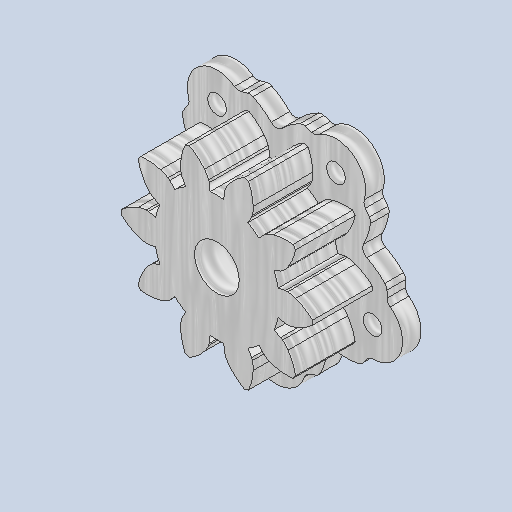
# Autodesk Inventor part: m2z10t8
Saved by Autodesk Inventor 2023 (Build 270158030, 158C)
## iProperties
Created: 2022-06-25
Part Number: m2z10t8
Material: アルミニウム 7075
Document SubType Name: Modeling
Designer: muzho
Density: 2.81 g/cm^3
Appearance: サテン - ブラシ仕上げ 重厚
Mass: 12.0512 g
Surface Area: 29.3851 cm^2
Volume: 4.2887 cm^3
Author: muzho
Autodesk Inventor part; units mm, degrees
ref_plane "YZ Plane" through (0, 0, 0) normal (1, 0, 0) x (0, 1, 0)
ref_plane "XZ Plane" through (0, 0, 0) normal (0, 1, 0) x (-1, 0, 0)
ref_plane "XY Plane" through (0, 0, 0) normal (0, 0, 1) x (1, 0, 0)
sketch "スケッチ3" plane through (0, 0, 0) normal (0, 0, 1) x (1, 0, 0)
  arc A0 (1.1108, 9.6353) -> (1.0261, 9.3407) centre (2.3523, 9.119) ccw
  arc A1 (1.6629, 10.5811) -> (1.1108, 9.6353) centre (4.6273, 8.2165) ccw
  arc A2 (3.6967, 12.3097) -> (1.6629, 10.5811) centre (7.0908, 6.2556) ccw
  arc A3 (-4.7648, 8.448) -> (-4.6602, 8.16) centre (-3.4569, 8.7601) ccw
  arc A4 (-4.8741, 9.5378) -> (-4.7648, 8.448) centre (-1.0859, 9.3672) ccw
  arc A5 (-4.2448, 12.1316) -> (-4.8741, 9.5378) centre (2.0596, 9.2288) ccw
  arc A6 (-8.8205, 4.0339) -> (-8.5665, 3.8624) centre (-7.9458, 5.0551) ccw
  arc A7 (-9.5494, 4.8513) -> (-8.8205, 4.0339) centre (-6.3844, 6.9399) ccw
  arc A8 (-10.5649, 7.3197) -> (-9.5494, 4.8513) centre (-3.7583, 8.6769) ccw
  arc A9 (-9.507, -1.921) -> (-9.2007, -1.9105) centre (-9.3996, -0.5807) ccw
  arc A10 (-10.5771, -1.6882) -> (-9.507, -1.921) centre (-9.2443, 1.8618) ccw
  arc A11 (-12.8496, -0.2881) -> (-10.5771, -1.6882) centre (-8.1406, 4.8107) ccw
  arc A12 (-6.5621, -7.1422) -> (-6.3205, -6.9537) centre (-7.2631, -5.9948) ccw
  arc A13 (-7.5648, -7.5828) -> (-6.5621, -7.1422) centre (-8.5731, -3.9274) ccw
  arc A14 (-10.2262, -7.7859) -> (-7.5648, -7.5828) centre (-9.4136, -0.893) ccw
  arc A15 (-1.1108, -9.6353) -> (-1.0261, -9.3407) centre (-2.3523, -9.119) ccw
  arc A16 (-1.6629, -10.5811) -> (-1.1108, -9.6353) centre (-4.6273, -8.2165) ccw
  arc A17 (-3.6967, -12.3097) -> (-1.6629, -10.5811) centre (-7.0908, -6.2556) ccw
  arc A18 (4.7648, -8.448) -> (4.6602, -8.16) centre (3.4569, -8.7601) ccw
  arc A19 (4.8741, -9.5378) -> (4.7648, -8.448) centre (1.0859, -9.3672) ccw
  arc A20 (4.2448, -12.1316) -> (4.8741, -9.5378) centre (-2.0596, -9.2288) ccw
  arc A21 (8.8205, -4.0339) -> (8.5665, -3.8624) centre (7.9458, -5.0551) ccw
  arc A22 (9.5494, -4.8513) -> (8.8205, -4.0339) centre (6.3844, -6.9399) ccw
  arc A23 (10.5649, -7.3197) -> (9.5494, -4.8513) centre (3.7583, -8.6769) ccw
  arc A24 (9.507, 1.921) -> (9.2007, 1.9105) centre (9.3996, 0.5807) ccw
  arc A25 (10.5771, 1.6882) -> (9.507, 1.921) centre (9.2443, -1.8618) ccw
  arc A26 (12.8496, 0.2881) -> (10.5771, 1.6882) centre (8.1406, -4.8107) ccw
  arc A27 (6.5621, 7.1422) -> (6.3205, 6.9537) centre (7.2631, 5.9948) ccw
  arc A28 (7.5648, 7.5828) -> (6.5621, 7.1422) centre (8.5731, 3.9274) ccw
  arc A29 (10.2262, 7.7859) -> (7.5648, 7.5828) centre (9.4136, 0.893) ccw
  arc A30 (-1.0261, 9.3407) -> (-1.1108, 9.6353) centre (-2.3523, 9.119) ccw
  arc A31 (-1.1108, 9.6353) -> (-1.6629, 10.5811) centre (-4.6273, 8.2165) ccw
  arc A32 (-1.6629, 10.5811) -> (-3.6967, 12.3097) centre (-7.0908, 6.2556) ccw
  arc A33 (-6.3205, 6.9537) -> (-6.5621, 7.1422) centre (-7.2631, 5.9948) ccw
  arc A34 (-6.5621, 7.1422) -> (-7.5648, 7.5828) centre (-8.5731, 3.9274) ccw
  arc A35 (-7.5648, 7.5828) -> (-10.2262, 7.7859) centre (-9.4136, 0.893) ccw
  arc A36 (-9.2007, 1.9105) -> (-9.507, 1.921) centre (-9.3996, 0.5807) ccw
  arc A37 (-9.507, 1.921) -> (-10.5771, 1.6882) centre (-9.2443, -1.8618) ccw
  arc A38 (-10.5771, 1.6882) -> (-12.8496, 0.2881) centre (-8.1406, -4.8107) ccw
  arc A39 (-8.5665, -3.8624) -> (-8.8205, -4.0339) centre (-7.9458, -5.0551) ccw
  arc A40 (-8.8205, -4.0339) -> (-9.5494, -4.8513) centre (-6.3844, -6.9399) ccw
  arc A41 (-9.5494, -4.8513) -> (-10.5649, -7.3197) centre (-3.7583, -8.6769) ccw
  arc A42 (-4.6602, -8.16) -> (-4.7648, -8.448) centre (-3.4569, -8.7601) ccw
  arc A43 (-4.7648, -8.448) -> (-4.8742, -9.5338) centre (-1.0859, -9.3672) ccw
  arc A44 (-4.8742, -9.5338) -> (-4.2448, -12.1316) centre (2.0596, -9.2288) ccw
  arc A45 (1.0261, -9.3407) -> (1.1108, -9.6353) centre (2.3523, -9.119) ccw
  arc A46 (1.1108, -9.6353) -> (1.6629, -10.5811) centre (4.6273, -8.2165) ccw
  arc A47 (1.6629, -10.5811) -> (3.6967, -12.3097) centre (7.0908, -6.2556) ccw
  arc A48 (6.3205, -6.9537) -> (6.5621, -7.1422) centre (7.2631, -5.9948) ccw
  arc A49 (6.5621, -7.1422) -> (7.5648, -7.5828) centre (8.5731, -3.9274) ccw
  arc A50 (7.5648, -7.5828) -> (10.2262, -7.7859) centre (9.4136, -0.893) ccw
  arc A51 (9.2007, -1.9105) -> (9.507, -1.921) centre (9.3996, -0.5807) ccw
  arc A52 (9.507, -1.921) -> (10.5771, -1.6882) centre (9.2443, 1.8618) ccw
  arc A53 (10.5771, -1.6882) -> (12.8496, -0.2881) centre (8.1406, 4.8107) ccw
  arc A54 (8.5665, 3.8624) -> (8.8205, 4.0339) centre (7.9458, 5.0551) ccw
  arc A55 (8.8205, 4.0339) -> (9.5494, 4.8513) centre (6.3844, 6.9399) ccw
  arc A56 (9.5494, 4.8513) -> (10.5649, 7.3197) centre (3.7583, 8.6769) ccw
  arc A57 (4.6602, 8.16) -> (4.7648, 8.448) centre (3.4569, 8.7601) ccw
  arc A58 (4.7648, 8.448) -> (4.8741, 9.5378) centre (1.0859, 9.3672) ccw
  arc A59 (4.8741, 9.5378) -> (4.2448, 12.1316) centre (-2.0596, 9.2288) ccw
  arc A60 (0.9173, 8.3498) -> (-0.9173, 8.3498) centre (0, 0) ccw
  arc A61 (-4.1658, 7.2943) -> (-5.65, 6.2159) centre (0, 0) ccw
  arc A62 (-7.6576, 3.4526) -> (-8.2246, 1.7078) centre (0, 0) ccw
  arc A63 (-8.2246, -1.7078) -> (-7.6576, -3.4526) centre (0, 0) ccw
  arc A64 (-5.65, -6.2159) -> (-4.1658, -7.2943) centre (0, 0) ccw
  arc A65 (-0.9173, -8.3498) -> (0.9173, -8.3498) centre (0, 0) ccw
  arc A66 (4.1658, -7.2943) -> (5.65, -6.2159) centre (0, 0) ccw
  arc A67 (7.6576, -3.4526) -> (8.2246, -1.7078) centre (0, 0) ccw
  arc A68 (8.2246, 1.7078) -> (7.6576, 3.4526) centre (0, 0) ccw
  arc A69 (5.65, 6.2159) -> (4.1658, 7.2943) centre (0, 0) ccw
  arc A70 (-3.6967, 12.3097) -> (-4.2448, 12.1316) centre (0, 0) ccw
  arc A71 (-10.2262, 7.7859) -> (-10.5649, 7.3197) centre (0, 0) ccw
  arc A72 (-12.8496, 0.2881) -> (-12.8496, -0.2881) centre (0, 0) ccw
  arc A73 (-10.5649, -7.3197) -> (-10.2262, -7.7859) centre (0, 0) ccw
  arc A74 (-4.2448, -12.1316) -> (-3.6967, -12.3097) centre (0, 0) ccw
  arc A75 (3.6967, -12.3097) -> (4.2448, -12.1316) centre (0, 0) ccw
  arc A76 (10.2262, -7.7859) -> (10.5649, -7.3197) centre (0, 0) ccw
  arc A77 (12.8496, -0.2881) -> (12.8496, 0.2881) centre (0, 0) ccw
  arc A78 (10.5649, 7.3197) -> (10.2262, 7.7859) centre (0, 0) ccw
  arc A79 (4.2448, 12.1316) -> (3.6967, 12.3097) centre (0, 0) ccw
  line L0 (0.9173, 8.3498) -> (1.0261, 9.3407)
  line L1 (-4.1658, 7.2943) -> (-4.6602, 8.16)
  line L2 (-7.6576, 3.4526) -> (-8.5665, 3.8624)
  line L3 (-8.2246, -1.7078) -> (-9.2007, -1.9105)
  line L4 (-5.65, -6.2159) -> (-6.3205, -6.9537)
  line L5 (-0.9173, -8.3498) -> (-1.0261, -9.3407)
  line L6 (4.1658, -7.2943) -> (4.6602, -8.16)
  line L7 (7.6576, -3.4526) -> (8.5665, -3.8624)
  line L8 (8.2246, 1.7078) -> (9.2007, 1.9105)
  line L9 (5.65, 6.2159) -> (6.3205, 6.9537)
  line L10 (-0.9173, 8.3498) -> (-1.0261, 9.3407)
  line L11 (-5.65, 6.2159) -> (-6.3205, 6.9537)
  line L12 (-8.2246, 1.7078) -> (-9.2007, 1.9105)
  line L13 (-7.6576, -3.4526) -> (-8.5665, -3.8624)
  line L14 (-4.1658, -7.2943) -> (-4.6602, -8.16)
  line L15 (0.9173, -8.3498) -> (1.0261, -9.3407)
  line L16 (5.65, -6.2159) -> (6.3205, -6.9537)
  line L17 (8.2246, -1.7078) -> (9.2007, -1.9105)
  line L18 (7.6576, 3.4526) -> (8.5665, 3.8624)
  line L19 (4.1658, 7.2943) -> (4.6602, 8.16)
  circle A80 centre (0, 0) radius 3
  point P0 (0, 0)
  dimension "d3" = 6
  constraints: 160 point on circle, 81 centre point, 40 end point, 1 coincident
  measures "d3" diameter of A80
extrude "押し出し2" add sketch "スケッチ3" along normal blind 8
sketch "スケッチ4" plane through (0, 0, 0) normal (0, 0, -1) x (-1, 0, 0)
  line L0 (-4.1658, 7.2943) -> (-4.6602, 8.16) projected
  arc A0 (-4.1658, 7.2943) -> (-5.65, 6.2159) centre (0, 0) ccw projected
  line L1 (-6.3205, 6.9537) -> (-5.65, 6.2159) projected
  arc A1 (-6.3205, 6.9537) -> (-6.5621, 7.1422) centre (-7.2631, 5.9948) ccw projected
  arc A2 (-6.5621, 7.1422) -> (-7.5648, 7.5828) centre (-8.5731, 3.9274) ccw projected
  arc A3 (-7.5648, 7.5828) -> (-10.2262, 7.7859) centre (-9.4136, 0.893) ccw projected
  arc A4 (-10.2262, 7.7859) -> (-10.5649, 7.3197) centre (0, 0) ccw projected
  arc A5 (-10.5649, 7.3197) -> (-9.5494, 4.8513) centre (-3.7583, 8.6769) ccw projected
  arc A6 (-9.5494, 4.8513) -> (-8.8205, 4.0339) centre (-6.3844, 6.9399) ccw projected
  arc A7 (-8.8205, 4.0339) -> (-8.5665, 3.8624) centre (-7.9458, 5.0551) ccw projected
  line L2 (-7.6576, 3.4526) -> (-8.5665, 3.8624) projected
  arc A8 (-7.6576, 3.4526) -> (-8.2246, 1.7078) centre (0, 0) ccw projected
  line L3 (-9.2007, 1.9105) -> (-8.2246, 1.7078) projected
  arc A9 (-9.2007, 1.9105) -> (-9.507, 1.921) centre (-9.3996, 0.5807) ccw projected
  arc A10 (-9.507, 1.921) -> (-10.5771, 1.6882) centre (-9.2443, -1.8618) ccw projected
  arc A11 (-10.5771, 1.6882) -> (-12.8496, 0.2881) centre (-8.1406, -4.8107) ccw projected
  arc A12 (-12.8496, 0.2881) -> (-12.8496, -0.2881) centre (0, 0) ccw projected
  arc A13 (-12.8496, -0.2881) -> (-10.5771, -1.6882) centre (-8.1406, 4.8107) ccw projected
  arc A14 (-10.5771, -1.6882) -> (-9.507, -1.921) centre (-9.2443, 1.8618) ccw projected
  arc A15 (-9.507, -1.921) -> (-9.2007, -1.9105) centre (-9.3996, -0.5807) ccw projected
  line L4 (-8.2246, -1.7078) -> (-9.2007, -1.9105) projected
  arc A16 (-8.2246, -1.7078) -> (-7.6576, -3.4526) centre (0, 0) ccw projected
  line L5 (-8.5665, -3.8624) -> (-7.6576, -3.4526) projected
  arc A17 (-8.5665, -3.8624) -> (-8.8205, -4.0339) centre (-7.9458, -5.0551) ccw projected
  arc A18 (-8.8205, -4.0339) -> (-9.5494, -4.8513) centre (-6.3844, -6.9399) ccw projected
  arc A19 (-9.5494, -4.8513) -> (-10.5649, -7.3197) centre (-3.7583, -8.6769) ccw projected
  arc A20 (-10.5649, -7.3197) -> (-10.2262, -7.7859) centre (0, 0) ccw projected
  arc A21 (-10.2262, -7.7859) -> (-7.5648, -7.5828) centre (-9.4136, -0.893) ccw projected
  arc A22 (-7.5648, -7.5828) -> (-6.5621, -7.1422) centre (-8.5731, -3.9274) ccw projected
  arc A23 (-6.5621, -7.1422) -> (-6.3205, -6.9537) centre (-7.2631, -5.9948) ccw projected
  line L6 (-5.65, -6.2159) -> (-6.3205, -6.9537) projected
  arc A24 (-5.65, -6.2159) -> (-4.1658, -7.2943) centre (0, 0) ccw projected
  line L7 (-4.6602, -8.16) -> (-4.1658, -7.2943) projected
  arc A25 (-4.6602, -8.16) -> (-4.7648, -8.448) centre (-3.4569, -8.7601) ccw projected
  arc A26 (-4.7648, -8.448) -> (-4.8741, -9.5378) centre (-1.0859, -9.3672) ccw projected
  arc A27 (-4.8741, -9.5378) -> (-4.2448, -12.1316) centre (2.0596, -9.2288) ccw projected
  arc A28 (-4.2448, -12.1316) -> (-3.6967, -12.3097) centre (0, 0) ccw projected
  arc A29 (-3.6967, -12.3097) -> (-1.6629, -10.5811) centre (-7.0908, -6.2556) ccw projected
  arc A30 (-1.6629, -10.5811) -> (-1.1108, -9.6353) centre (-4.6273, -8.2165) ccw projected
  arc A31 (-1.1108, -9.6353) -> (-1.0261, -9.3407) centre (-2.3523, -9.119) ccw projected
  line L8 (-0.9173, -8.3498) -> (-1.0261, -9.3407) projected
  arc A32 (-0.9173, -8.3498) -> (0.9173, -8.3498) centre (0, 0) ccw projected
  line L9 (1.0261, -9.3407) -> (0.9173, -8.3498) projected
  arc A33 (1.0261, -9.3407) -> (1.1108, -9.6353) centre (2.3523, -9.119) ccw projected
  arc A34 (1.1108, -9.6353) -> (1.6629, -10.5811) centre (4.6273, -8.2165) ccw projected
  arc A35 (1.6629, -10.5811) -> (3.6967, -12.3097) centre (7.0908, -6.2556) ccw projected
  arc A36 (3.6967, -12.3097) -> (4.2448, -12.1316) centre (0, 0) ccw projected
  arc A37 (4.2448, -12.1316) -> (4.8742, -9.5338) centre (-2.0596, -9.2288) ccw projected
  arc A38 (4.8742, -9.5338) -> (4.7648, -8.448) centre (1.0859, -9.3672) ccw projected
  arc A39 (4.7648, -8.448) -> (4.6602, -8.16) centre (3.4569, -8.7601) ccw projected
  line L10 (4.1658, -7.2943) -> (4.6602, -8.16) projected
  arc A40 (4.1658, -7.2943) -> (5.65, -6.2159) centre (0, 0) ccw projected
  line L11 (6.3205, -6.9537) -> (5.65, -6.2159) projected
  arc A41 (6.3205, -6.9537) -> (6.5621, -7.1422) centre (7.2631, -5.9948) ccw projected
  arc A42 (6.5621, -7.1422) -> (7.5648, -7.5828) centre (8.5731, -3.9274) ccw projected
  arc A43 (7.5648, -7.5828) -> (10.2262, -7.7859) centre (9.4136, -0.893) ccw projected
  arc A44 (10.2262, -7.7859) -> (10.5649, -7.3197) centre (0, 0) ccw projected
  arc A45 (10.5649, -7.3197) -> (9.5494, -4.8513) centre (3.7583, -8.6769) ccw projected
  arc A46 (9.5494, -4.8513) -> (8.8205, -4.0339) centre (6.3844, -6.9399) ccw projected
  arc A47 (8.8205, -4.0339) -> (8.5665, -3.8624) centre (7.9458, -5.0551) ccw projected
  line L12 (7.6576, -3.4526) -> (8.5665, -3.8624) projected
  arc A48 (7.6576, -3.4526) -> (8.2246, -1.7078) centre (0, 0) ccw projected
  line L13 (9.2007, -1.9105) -> (8.2246, -1.7078) projected
  arc A49 (9.2007, -1.9105) -> (9.507, -1.921) centre (9.3996, -0.5807) ccw projected
  arc A50 (9.507, -1.921) -> (10.5771, -1.6882) centre (9.2443, 1.8618) ccw projected
  arc A51 (10.5771, -1.6882) -> (12.8496, -0.2881) centre (8.1406, 4.8107) ccw projected
  arc A52 (12.8496, -0.2881) -> (12.8496, 0.2881) centre (0, 0) ccw projected
  arc A53 (12.8496, 0.2881) -> (10.5771, 1.6882) centre (8.1406, -4.8107) ccw projected
  arc A54 (10.5771, 1.6882) -> (9.507, 1.921) centre (9.2443, -1.8618) ccw projected
  arc A55 (9.507, 1.921) -> (9.2007, 1.9105) centre (9.3996, 0.5807) ccw projected
  line L14 (8.2246, 1.7078) -> (9.2007, 1.9105) projected
  arc A56 (8.2246, 1.7078) -> (7.6576, 3.4526) centre (0, 0) ccw projected
  line L15 (8.5665, 3.8624) -> (7.6576, 3.4526) projected
  arc A57 (8.5665, 3.8624) -> (8.8205, 4.0339) centre (7.9458, 5.0551) ccw projected
  arc A58 (8.8205, 4.0339) -> (9.5494, 4.8513) centre (6.3844, 6.9399) ccw projected
  arc A59 (9.5494, 4.8513) -> (10.5649, 7.3197) centre (3.7583, 8.6769) ccw projected
  arc A60 (10.5649, 7.3197) -> (10.2262, 7.7859) centre (0, 0) ccw projected
  arc A61 (10.2262, 7.7859) -> (7.5648, 7.5828) centre (9.4136, 0.893) ccw projected
  arc A62 (7.5648, 7.5828) -> (6.5621, 7.1422) centre (8.5731, 3.9274) ccw projected
  arc A63 (6.5621, 7.1422) -> (6.3205, 6.9537) centre (7.2631, 5.9948) ccw projected
  line L16 (5.65, 6.2159) -> (6.3205, 6.9537) projected
  arc A64 (5.65, 6.2159) -> (4.1658, 7.2943) centre (0, 0) ccw projected
  line L17 (4.6602, 8.16) -> (4.1658, 7.2943) projected
  arc A65 (4.6602, 8.16) -> (4.7648, 8.448) centre (3.4569, 8.7601) ccw projected
  arc A66 (4.7648, 8.448) -> (4.8741, 9.5378) centre (1.0859, 9.3672) ccw projected
  arc A67 (4.8741, 9.5378) -> (4.2448, 12.1316) centre (-2.0596, 9.2288) ccw projected
  arc A68 (4.2448, 12.1316) -> (3.6967, 12.3097) centre (0, 0) ccw projected
  arc A69 (3.6967, 12.3097) -> (1.6629, 10.5811) centre (7.0908, 6.2556) ccw projected
  arc A70 (1.6629, 10.5811) -> (1.1108, 9.6353) centre (4.6273, 8.2165) ccw projected
  arc A71 (1.1108, 9.6353) -> (1.0261, 9.3407) centre (2.3523, 9.119) ccw projected
  line L18 (0.9173, 8.3498) -> (1.0261, 9.3407) projected
  arc A72 (0.9173, 8.3498) -> (-0.9173, 8.3498) centre (0, 0) ccw projected
  line L19 (-1.0261, 9.3407) -> (-0.9173, 8.3498) projected
  arc A73 (-1.0261, 9.3407) -> (-1.1108, 9.6353) centre (-2.3523, 9.119) ccw projected
  arc A74 (-1.1108, 9.6353) -> (-1.6629, 10.5811) centre (-4.6273, 8.2165) ccw projected
  arc A75 (-1.6629, 10.5811) -> (-3.6967, 12.3097) centre (-7.0908, 6.2556) ccw projected
  arc A76 (-3.6967, 12.3097) -> (-4.2448, 12.1316) centre (0, 0) ccw projected
  arc A77 (-4.2448, 12.1316) -> (-4.8741, 9.5378) centre (2.0596, 9.2288) ccw projected
  arc A78 (-4.8741, 9.5378) -> (-4.7648, 8.448) centre (-1.0859, 9.3672) ccw projected
  arc A79 (-4.7648, 8.448) -> (-4.6602, 8.16) centre (-3.4569, 8.7601) ccw projected
  circle A80 centre (0, 0) radius 3 projected
  circle A81 centre (7.979, 10.9821) radius 1.25
  circle A82 centre (7.979, 10.9821) radius 4
  arc A83 (6.8778, 9.4665) -> (5.6653, 13.7299) centre (-2.0596, 9.2288) ccw
  arc A84 (5.65, 6.2159) -> (4.1658, 7.2943) centre (0, 0) ccw projected
  circle A85 centre (-7.979, 10.9821) radius 4
  circle A86 centre (-7.979, 10.9821) radius 1.25
  circle A87 centre (-12.9103, -4.1948) radius 4
  circle A88 centre (-12.9103, -4.1948) radius 1.25
  circle A89 centre (0, -13.5747) radius 4
  circle A90 centre (0, -13.5747) radius 1.25
  circle A91 centre (12.9103, -4.1948) radius 4
  circle A92 centre (12.9103, -4.1948) radius 1.25
  arc A93 (5.6653, 13.7299) -> (3.4869, 14.4377) centre (0, 0) ccw
  arc A94 (3.4869, 14.4377) -> (0, 11.7012) centre (7.0908, 6.2556) ccw
  arc A95 (-5.6653, 13.7299) -> (-6.8778, 9.4665) centre (2.0596, 9.2288) ccw
  arc A96 (-3.4869, 14.4377) -> (-5.6653, 13.7299) centre (0, 0) ccw
  arc A97 (0, 11.7012) -> (-3.4869, 14.4377) centre (-7.0908, 6.2556) ccw
  arc A98 (-12.6535, 7.7778) -> (-11.1285, 3.6159) centre (-3.7583, 8.6769) ccw
  arc A99 (-11.3073, 9.6308) -> (-12.6535, 7.7778) centre (0, 0) ccw
  arc A100 (-6.8778, 9.4665) -> (-11.3073, 9.6308) centre (-9.4136, 0.893) ccw
  arc A101 (-14.8086, -1.1452) -> (-11.1285, -3.6159) centre (-8.1406, 4.8107) ccw
  arc A102 (-14.8086, 1.1452) -> (-14.8086, -1.1452) centre (0, 0) ccw
  arc A103 (-11.1285, 3.6159) -> (-14.8086, 1.1452) centre (-8.1406, -4.8107) ccw
  arc A104 (-11.3073, -9.6308) -> (-6.8778, -9.4665) centre (-9.4136, -0.893) ccw
  arc A105 (-12.6535, -7.7778) -> (-11.3073, -9.6308) centre (0, 0) ccw
  arc A106 (-11.1285, -3.6159) -> (-12.6535, -7.7778) centre (-3.7583, -8.6769) ccw
  arc A107 (-3.4869, -14.4377) -> (0, -11.7012) centre (-7.0908, -6.2556) ccw
  arc A108 (-5.6653, -13.7299) -> (-3.4869, -14.4377) centre (0, 0) ccw
  arc A109 (-6.8778, -9.4665) -> (-5.6653, -13.7299) centre (2.0596, -9.2288) ccw
  arc A110 (5.6653, -13.7299) -> (6.8778, -9.4665) centre (-2.0596, -9.2288) ccw
  arc A111 (3.4869, -14.4377) -> (5.6653, -13.7299) centre (0, 0) ccw
  arc A112 (0, -11.7012) -> (3.4869, -14.4377) centre (7.0908, -6.2556) ccw
  arc A113 (12.6535, -7.7778) -> (11.1285, -3.6159) centre (3.7583, -8.6769) ccw
  arc A114 (11.3073, -9.6308) -> (12.6535, -7.7778) centre (0, 0) ccw
  arc A115 (6.8778, -9.4665) -> (11.3073, -9.6308) centre (9.4136, -0.893) ccw
  arc A116 (14.8086, 1.1452) -> (11.1285, 3.6159) centre (8.1406, -4.8107) ccw
  arc A117 (14.8086, -1.1452) -> (14.8086, 1.1452) centre (0, 0) ccw
  arc A118 (11.1285, -3.6159) -> (14.8086, -1.1452) centre (8.1406, 4.8107) ccw
  arc A119 (11.3073, 9.6308) -> (6.8778, 9.4665) centre (9.4136, 0.893) ccw
  arc A120 (12.6535, 7.7778) -> (11.3073, 9.6308) centre (0, 0) ccw
  arc A121 (11.1285, 3.6159) -> (12.6535, 7.7778) centre (3.7583, 8.6769) ccw
  point P0 (-11.5981, 9.2785)
  point P1 (-11.1285, 3.6159)
  point P2 (-14.8368, -0.6893)
  point P3 (-12.4084, -8.1632)
  point P4 (-6.8778, -9.4665)
  point P5 (-3.9293, -14.3236)
  point P6 (3.9293, -14.3236)
  point P7 (6.8778, -9.4665)
  point P8 (12.4084, -8.1632)
  point P9 (14.8368, -0.6893)
  point P10 (11.1285, 3.6159)
  point P11 (11.5981, 9.2785)
  point P12 (5.2404, 13.8976)
  point P13 (-5.2404, 13.8976)
  dimension "d6" = 2.5
  dimension "d7" = 8
  dimension "d8" = 2
  dimension "d11" = 360
  dimension "d13" = 2
  dimension "d14" = 2
  dimension "d17" = 360
  constraints: 61 point on circle, 40 centre point, 6 coincident, 3 concentric, 2 tangent, 122 other
  measures "d6" diameter of A81
  measures "d7" diameter of A82
  measures "d8" radial gap between concentric circles of A67 A83
  measures "d13" radial gap between concentric circles of A68 A93
  measures "d14" radial gap between concentric circles of A69 A94
extrude "押し出し3" add sketch "スケッチ4" along normal blind 2.5 contours A0 L1 A1 A2 A85 A78 A79 L0 | L0 A79 A78 A85 A76 A75 A74 A73 L19 A72 L18 A71 A70 A69 A68 A82 A66 A65 L17 A64 L16 A63 A62 A60 A59 A58 A57 L15 A56 L14 A55 A54 A53 A52 A91 A50 A49 L13 A48 L12 A47 A46 A44 A43 A42 A41 L11 A40 L10 A39 A38 A37 A36 A89 A34 A33 L9 A32 L8 A31 A30 A28 A27 A26 A25 L7 A24 L6 A23 A22 A21 A20 A87 A18 A17 L5 A16 L4 A15 A14 A12 A11 A10 A9 L3 A8 L2 A7 A6 A5 A4 A2 A1 L1 A0 | A85 A2 A3 A4 A99 A100 A95 A96 A76 A77 A78 | A78 A77 A76 A85 | A85 A4 A3 A2 | A4 A5 A6 A7 L2 A8 L3 A9 A10 A11 A12 A87 A102 A103 A98 A99 A85 | A85 A96 A97 A94 A93 A82 A68 A69 A70 A71 L18 A72 L19 A73 A74 A75 A76 | A85 A96 A95 A86 A100 A99 | A86 A95 A100 | A102 A101 A88 A106 A105 A87 | A87 A12 A13 A14 A18 A19 A20 A105 A106 A101 A102 | A93 A83 A119 A120 A82 A60 A61 A62 A66 A67 A68 | A82 A120 A119 A81 A83 A93 | A87 A14 A13 A12 | A87 A20 A21 A22 A23 L6 A24 L7 A25 A26 A27 A28 A89 A108 A109 A104 A105 | A68 A67 A66 A82 | A14 A15 L4 A16 L5 A17 A18 A87 | A20 A19 A18 A87 | A101 A106 A88 | A120 A121 A116 A117 A91 A52 A53 A54 A55 L14 A56 L15 A57 A58 A59 A60 A82 | A82 A62 A63 L16 A64 L17 A65 A66 | A81 A119 A83 | A82 A62 A61 A60 | A108 A107 A90 A112 A111 A89 | A89 A28 A29 A30 A34 A35 A36 A111 A112 A107 A108 | A89 A30 A29 A28 | A89 A36 A37 A38 A39 L10 A40 L11 A41 A42 A43 A44 A91 A114 A115 A110 A111 | A117 A118 A113 A114 A91 A44 A45 A46 A50 A51 A52 | A91 A114 A113 A92 A118 A117 | A30 A31 L8 A32 L9 A33 A34 A89 | A107 A112 A90 | A52 A51 A50 A91 | A89 A36 A35 A34 | A91 A46 A47 L12 A48 L13 A49 A50 | A92 A113 A118 | A91 A46 A45 A44
fillet "フィレット1" radius 1 25 edges at (11.5981, 9.2785, -1.25) (12.6535, 7.7778, -1.25) (11.1285, 3.6159, -1.25) (14.8086, 1.1452, -1.25) (14.8368, -0.6893, -1.25) (12.4084, -8.1632, -1.25) (11.3073, -9.6308, -1.25) (6.8778, -9.4665, -1.25) (5.6653, -13.7299, -1.25) (3.9293, -14.3236, -1.25) (-3.9293, -14.3236, -1.25) (-5.6653, -13.7299, -1.25) (-6.8778, -9.4665, -1.25) (-11.3073, -9.6308, -1.25) (-12.4084, -8.1632, -1.25) (-14.8368, -0.6893, -1.25) (-14.8086, 1.1452, -1.25) (-11.1285, 3.6159, -1.25) (-12.6535, 7.7778, -1.25) (-11.5981, 9.2785, -1.25) (-5.2404, 13.8976, -1.25) (-3.4869, 14.4377, -1.25) (0, 11.7012, -1.25) (3.4869, 14.4377, -1.25) (5.2404, 13.8976, -1.25)
sketch "スケッチ5" plane through (0, 0, -2.5) normal (0, 0, -1) x (-1, 0, 0)
  arc A0 (-3.1442, 14.278) -> (-3.8445, 14.3466) centre (-3.5856, 13.3807) ccw projected
  arc A1 (-3.8445, 14.3466) -> (-4.7248, 14.0812) centre (0, 0) ccw projected
  arc A2 (-5.6301, 14.2199) -> (-4.7248, 14.0812) centre (-5.0429, 15.0293) ccw projected
  arc A3 (-5.6301, 14.2199) -> (-11.7841, 9.7488) centre (-7.979, 10.9821) ccw projected
  arc A4 (-11.932, 8.8449) -> (-11.7841, 9.7488) centre (-12.7354, 9.4404) ccw projected
  arc A5 (-11.932, 8.8449) -> (-12.4564, 8.0897) centre (0, 0) ccw projected
  arc A6 (-12.4564, 8.0897) -> (-12.6076, 7.4025) centre (-11.6178, 7.545) ccw projected
  arc A7 (-12.6076, 7.4025) -> (-11.6883, 4.5478) centre (-3.7583, 8.6769) ccw projected
  arc A8 (-12.1291, 3.191) -> (-11.6883, 4.5478) centre (-12.5752, 4.0859) ccw projected
  arc A9 (-12.1291, 3.191) -> (-14.5508, 1.4218) centre (-8.1406, -4.8107) ccw projected
  arc A10 (-14.5508, 1.4218) -> (-14.8325, 0.777) centre (-13.8338, 0.7247) ccw projected
  arc A11 (-14.8325, 0.777) -> (-14.8521, -0.1422) centre (0, 0) ccw projected
  arc A12 (-15.2637, -0.9604) -> (-14.8521, -0.1422) centre (-15.8521, -0.1518) ccw projected
  arc A13 (-15.2637, -0.9604) -> (-12.9131, -8.1948) centre (-12.9103, -4.1948) ccw projected
  arc A14 (-12.0992, -8.6148) -> (-12.9131, -8.1948) centre (-12.9138, -9.1948) ccw projected
  arc A15 (-12.0992, -8.6148) -> (-11.543, -9.3469) centre (0, 0) ccw projected
  arc A16 (-11.543, -9.3469) -> (-10.9361, -9.703) centre (-10.7658, -8.7176) ccw projected
  arc A17 (-10.9361, -9.703) -> (-7.9371, -9.7108) centre (-9.4136, -0.893) ccw projected
  arc A18 (-6.7829, -10.5494) -> (-7.9371, -9.7108) centre (-7.7719, -10.6971) ccw projected
  arc A19 (-6.7829, -10.5494) -> (-5.8487, -13.3993) centre (2.0596, -9.2288) ccw projected
  arc A20 (-5.8487, -13.3993) -> (-5.3225, -13.8664) centre (-4.9641, -12.9328) ccw projected
  arc A21 (-5.3225, -13.8664) -> (-4.4543, -14.1692) centre (0, 0) ccw projected
  arc A22 (-3.8033, -14.8134) -> (-4.4543, -14.1692) centre (-4.7542, -15.1231) ccw projected
  arc A23 (-3.8033, -14.8134) -> (3.8033, -14.8134) centre (0, -13.5747) ccw projected
  arc A24 (4.4543, -14.1692) -> (3.8033, -14.8134) centre (4.7542, -15.1231) ccw projected
  arc A25 (4.4543, -14.1692) -> (5.3225, -13.8664) centre (0, 0) ccw projected
  arc A26 (5.3225, -13.8664) -> (5.8487, -13.3993) centre (4.9641, -12.9328) ccw projected
  arc A27 (5.8487, -13.3993) -> (6.7829, -10.5494) centre (-2.0596, -9.2288) ccw projected
  arc A28 (7.9371, -9.7108) -> (6.7829, -10.5494) centre (7.7719, -10.6971) ccw projected
  arc A29 (7.9371, -9.7108) -> (10.9361, -9.703) centre (9.4136, -0.893) ccw projected
  arc A30 (10.9361, -9.703) -> (11.543, -9.3469) centre (10.7658, -8.7176) ccw projected
  arc A31 (11.543, -9.3469) -> (12.0992, -8.6148) centre (0, 0) ccw projected
  arc A32 (12.9131, -8.1948) -> (12.0992, -8.6148) centre (12.9138, -9.1948) ccw projected
  arc A33 (12.9131, -8.1948) -> (15.2637, -0.9604) centre (12.9103, -4.1948) ccw projected
  arc A34 (14.8521, -0.1422) -> (15.2637, -0.9604) centre (15.8521, -0.1518) ccw projected
  arc A35 (14.8521, -0.1422) -> (14.8325, 0.777) centre (0, 0) ccw projected
  arc A36 (14.8325, 0.777) -> (14.5508, 1.4218) centre (13.8338, 0.7247) ccw projected
  arc A37 (14.5508, 1.4218) -> (12.1291, 3.191) centre (8.1406, -4.8107) ccw projected
  arc A38 (11.6883, 4.5478) -> (12.1291, 3.191) centre (12.5752, 4.0859) ccw projected
  arc A39 (11.6883, 4.5478) -> (12.6076, 7.4025) centre (3.7583, 8.6769) ccw projected
  arc A40 (12.6076, 7.4025) -> (12.4564, 8.0897) centre (11.6178, 7.545) ccw projected
  arc A41 (12.4564, 8.0897) -> (11.932, 8.8449) centre (0, 0) ccw projected
  arc A42 (11.7841, 9.7488) -> (11.932, 8.8449) centre (12.7354, 9.4404) ccw projected
  arc A43 (11.7841, 9.7488) -> (5.6301, 14.2199) centre (7.979, 10.9821) ccw projected
  arc A44 (4.7248, 14.0812) -> (5.6301, 14.2199) centre (5.0429, 15.0293) ccw projected
  arc A45 (4.7248, 14.0812) -> (3.8445, 14.3466) centre (0, 0) ccw projected
  arc A46 (3.8445, 14.3466) -> (3.1442, 14.278) centre (3.5856, 13.3807) ccw projected
  arc A47 (3.1442, 14.278) -> (0.7133, 12.5215) centre (7.0908, 6.2556) ccw projected
  arc A48 (-0.7133, 12.5215) -> (0.7133, 12.5215) centre (0, 13.2224) ccw projected
  arc A49 (-0.7133, 12.5215) -> (-3.1442, 14.278) centre (-7.0908, 6.2556) ccw projected
  circle A50 centre (-7.979, 10.9821) radius 1.25 projected
  circle A51 centre (12.9103, -4.1948) radius 1.25 projected
  circle A52 centre (-12.9103, -4.1948) radius 1.25 projected
  circle A53 centre (0, 0) radius 3 projected
  circle A54 centre (0, -13.5747) radius 1.25 projected
  circle A55 centre (7.979, 10.9821) radius 1.25 projected
